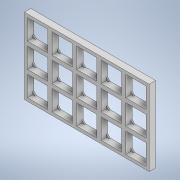
# Autodesk Inventor part: Cherry_Switch_Alignment_Jig
Saved by Autodesk Inventor 2022.2 (Build 262287000, 287)
## iProperties
Created: 2022-12-30
Part Number: Cherry_Switch_Alignment_Jig
Material: Generisch
Document SubType Name: Modeling
Designer: Frederik
Density: 1 g/cm^3
Appearance: Vorgabe
Author: Frederik
Autodesk Inventor part; units mm, degrees
ref_plane "YZ Plane" through (0, 0, 0) normal (1, 0, 0) x (0, 1, 0)
ref_plane "XZ Plane" through (0, 0, 0) normal (0, 1, 0) x (-1, 0, 0)
ref_plane "XY Plane" through (0, 0, 0) normal (0, 0, 1) x (1, 0, 0)
sketch "Skizze1" plane through (0, 0, 0) normal (0, 0, 1) x (1, 0, 0)
  line L0 (0, 0) -> (15.6, 0) construction
  line L1 (15.6, 0) -> (15.6, 15.6) construction
  line L2 (15.6, 15.6) -> (0, 15.6) construction
  line L3 (0, 15.6) -> (0, 0) construction
  line L4 (-0.09, 15.69) -> (15.69, 15.69)
  line L5 (15.69, 15.69) -> (15.69, -0.09)
  line L6 (15.69, -0.09) -> (-0.09, -0.09)
  line L7 (-0.09, -0.09) -> (-0.09, 15.69)
  line L8 (1.91, 15.69) -> (-0.09, 13.69)
  line L9 (13.69, 15.69) -> (15.69, 13.69)
  line L10 (15.69, 1.91) -> (13.69, -0.09)
  line L11 (1.91, -0.09) -> (-0.09, 1.91)
  line L12 (-0.09, -0.09) -> (15.69, 15.69) construction
  line L13 (15.69, -0.09) -> (-0.09, 15.69) construction
  line L14 (-1.725, 17.325) -> (17.325, 17.325)
  line L15 (17.325, 17.325) -> (17.325, -1.725)
  line L16 (17.325, -1.725) -> (-1.725, -1.725)
  line L17 (-1.725, -1.725) -> (-1.725, 17.325)
  point P0 (7.8, 7.8)
  point P1 (7.8, 7.8)
  dimension "d0" = 15.6
  dimension "d1" = 15.6
  dimension "d2" = 0.09
  dimension "d3" = 2
  dimension "d4" = 2
  dimension "d5" = 2
  dimension "d6" = 2
  dimension "d7" = 2
  dimension "d8" = 2
  dimension "d9" = 2
  dimension "d10" = 2
  dimension "d11" = 9.525
  constraints: 36 end point, 9 point on line, 6 parallel, 4 perpendicular, 2 midpoint, 1 horizontal, 6 other
  measures "d0" distance of L1.end L2.end
  measures "d1" distance of L0.end L1.end
  measures "d2" distance between parallel lines of L2 L4
  measures "d3" distance from line of L7 L8.start
  measures "d4" distance from line of L4 L8.end
  measures "d5" distance from line of L5 L9.start
  measures "d6" distance from line of L4 L9.end
  measures "d7" distance from line of L6 L10.start
  measures "d8" distance from line of L5 L10.end
  measures "d9" distance from line of L6 L11.end
  measures "d10" distance from line of L7 L11.start
  measures "d11" distance from line of L17 point (7.8, 7.8)
extrude "Extrusion1" add sketch "Skizze1" along normal blind 1 contours L4 L8 L7 | L4 L5 L9 | L11 L6 L7 | L5 L6 L10 | L14 L15 L16 L17
sketch "Skizze2" plane through (0, 0, 1) normal (0, 0, 1) x (1, 0, 0)
  line L0 (-1.725, -1.725) -> (17.325, -1.725) projected
  line L1 (17.325, -1.725) -> (17.325, 17.325) projected
  line L2 (17.325, 17.325) -> (-1.725, 17.325) projected
  line L3 (-1.725, 17.325) -> (-1.725, -1.725) projected
  line L4 (-0.09, 13.69) -> (1.91, 15.69) projected
  line L5 (1.91, 15.69) -> (13.69, 15.69) projected
  line L6 (13.69, 15.69) -> (15.69, 13.69) projected
  line L7 (15.69, 13.69) -> (15.69, 1.91) projected
  line L8 (15.69, 1.91) -> (13.69, -0.09) projected
  line L9 (13.69, -0.09) -> (1.91, -0.09) projected
  line L10 (1.91, -0.09) -> (-0.09, 1.91) projected
  line L11 (-0.09, 1.91) -> (-0.09, 13.69) projected
  line L12 (1.91, 15.69) -> (13.69, 15.69) projected
  line L13 (1.91, 15.69) -> (-0.09, 15.69)
  line L14 (-0.09, 15.69) -> (-0.09, 13.69)
  line L15 (-0.09, 1.91) -> (-0.09, 13.69) projected
  line L16 (-0.09, 1.91) -> (-0.09, -0.09)
  line L17 (-0.09, -0.09) -> (1.91, -0.09)
  line L18 (13.69, -0.09) -> (1.91, -0.09) projected
  line L19 (13.69, -0.09) -> (15.69, -0.09)
  line L20 (15.69, 1.91) -> (13.69, -0.09) projected
  line L21 (15.69, -0.09) -> (15.69, 1.91)
  line L22 (15.69, 13.69) -> (15.69, 1.91) projected
  line L23 (15.69, 13.69) -> (15.69, 15.69)
  line L24 (13.69, 15.69) -> (15.69, 13.69) projected
  line L25 (15.69, 15.69) -> (13.69, 15.69)
  point P0 (0, 0)
  constraints: 16 end point, 3 perpendicular, 3 point on line, 1 collinear, 1 vertical
extrude "Extrusion2" add sketch "Skizze2" along normal blind 4
pattern_linear "Rechteckige Anordnung1" count 5 spacing 19.05 along (1, 0, 0) count 3 spacing 19.05 along (0, -1, 0)
sketch "Skizze3" plane through (0, 0, 5) normal (0, 0, 1) x (1, 0, 0)
  line L0 (93.525, 17.325) -> (-1.725, 17.325) projected
  line L1 (-1.725, 17.325) -> (-1.725, -39.825) projected
  line L2 (-0.09, 15.69) -> (15.69, 15.69) projected
  line L3 (15.69, 15.69) -> (15.69, -0.09) projected
  line L4 (15.69, -0.09) -> (-0.09, -0.09) projected
  line L5 (-0.09, -0.09) -> (-0.09, 15.69) projected
  line L6 (-1.725, -39.825) -> (93.525, -39.825) projected
  line L7 (93.525, -39.825) -> (93.525, 17.325) projected
  line L8 (18.96, 15.69) -> (34.74, 15.69) projected
  line L9 (34.74, 15.69) -> (34.74, -0.09) projected
  line L10 (34.74, -0.09) -> (18.96, -0.09) projected
  line L11 (18.96, -0.09) -> (18.96, 15.69) projected
  line L12 (38.01, 15.69) -> (53.79, 15.69) projected
  line L13 (53.79, 15.69) -> (53.79, -0.09) projected
  line L14 (53.79, -0.09) -> (38.01, -0.09) projected
  line L15 (38.01, -0.09) -> (38.01, 15.69) projected
  line L16 (57.06, 15.69) -> (72.84, 15.69) projected
  line L17 (72.84, 15.69) -> (72.84, -0.09) projected
  line L18 (72.84, -0.09) -> (57.06, -0.09) projected
  line L19 (57.06, -0.09) -> (57.06, 15.69) projected
  line L20 (76.11, 15.69) -> (91.89, 15.69) projected
  line L21 (91.89, 15.69) -> (91.89, -0.09) projected
  line L22 (91.89, -0.09) -> (76.11, -0.09) projected
  line L23 (76.11, -0.09) -> (76.11, 15.69) projected
  line L24 (18.96, -3.36) -> (34.74, -3.36) projected
  line L25 (34.74, -3.36) -> (34.74, -19.14) projected
  line L26 (34.74, -19.14) -> (18.96, -19.14) projected
  line L27 (18.96, -19.14) -> (18.96, -3.36) projected
  line L28 (-0.09, -3.36) -> (15.69, -3.36) projected
  line L29 (15.69, -3.36) -> (15.69, -19.14) projected
  line L30 (15.69, -19.14) -> (-0.09, -19.14) projected
  line L31 (-0.09, -19.14) -> (-0.09, -3.36) projected
  line L32 (38.01, -3.36) -> (53.79, -3.36) projected
  line L33 (53.79, -3.36) -> (53.79, -19.14) projected
  line L34 (53.79, -19.14) -> (38.01, -19.14) projected
  line L35 (38.01, -19.14) -> (38.01, -3.36) projected
  line L36 (57.06, -3.36) -> (72.84, -3.36) projected
  line L37 (72.84, -3.36) -> (72.84, -19.14) projected
  line L38 (72.84, -19.14) -> (57.06, -19.14) projected
  line L39 (57.06, -19.14) -> (57.06, -3.36) projected
  line L40 (76.11, -3.36) -> (91.89, -3.36) projected
  line L41 (91.89, -3.36) -> (91.89, -19.14) projected
  line L42 (91.89, -19.14) -> (76.11, -19.14) projected
  line L43 (76.11, -19.14) -> (76.11, -3.36) projected
  line L44 (-0.09, -22.41) -> (15.69, -22.41) projected
  line L45 (15.69, -22.41) -> (15.69, -38.19) projected
  line L46 (15.69, -38.19) -> (-0.09, -38.19) projected
  line L47 (-0.09, -38.19) -> (-0.09, -22.41) projected
  line L48 (18.96, -22.41) -> (34.74, -22.41) projected
  line L49 (34.74, -22.41) -> (34.74, -38.19) projected
  line L50 (34.74, -38.19) -> (18.96, -38.19) projected
  line L51 (18.96, -38.19) -> (18.96, -22.41) projected
  line L52 (38.01, -22.41) -> (53.79, -22.41) projected
  line L53 (53.79, -22.41) -> (53.79, -38.19) projected
  line L54 (53.79, -38.19) -> (38.01, -38.19) projected
  line L55 (38.01, -38.19) -> (38.01, -22.41) projected
  line L56 (57.06, -22.41) -> (72.84, -22.41) projected
  line L57 (72.84, -22.41) -> (72.84, -38.19) projected
  line L58 (72.84, -38.19) -> (57.06, -38.19) projected
  line L59 (57.06, -38.19) -> (57.06, -22.41) projected
  line L60 (76.11, -22.41) -> (91.89, -22.41) projected
  line L61 (91.89, -22.41) -> (91.89, -38.19) projected
  line L62 (91.89, -38.19) -> (76.11, -38.19) projected
  line L63 (76.11, -38.19) -> (76.11, -22.41) projected
  line L64 (93.525, 17.325) -> (-1.725, 17.325) projected
  line L65 (-1.725, 17.325) -> (-1.725, -39.825) projected
  line L66 (-1.725, -39.825) -> (93.525, -39.825) projected
  line L67 (93.525, -39.825) -> (93.525, 17.325) projected
  line L68 (-0.09, 15.69) -> (15.69, 15.69) projected
  line L69 (15.69, 15.69) -> (15.69, -0.09) projected
  line L70 (15.69, -0.09) -> (-0.09, -0.09) projected
  line L71 (-0.09, -0.09) -> (-0.09, 15.69) projected
  line L72 (-2.49, 18.09) -> (94.29, 18.09)
  line L73 (94.29, 18.09) -> (94.29, -40.59)
  line L74 (94.29, -40.59) -> (-2.49, -40.59)
  line L75 (-2.49, -40.59) -> (-2.49, 18.09)
  dimension "d26" = 0.765
  constraints: 8 end point, 3 other
  measures "d26" distance between parallel lines of L0 L72
extrude "Extrusion3" add sketch "Skizze3" against normal up to surface (5 mm away) contours L72 L73 L74 L75
equation "\"d1\" = d0"
equation "\"d2\" = clearance"
equation "\"d3\" = dLength"
equation "\"d4\" = dLength"
equation "\"d5\" = dLength"
equation "\"d6\" = dLength"
equation "\"d7\" = dLength"
equation "\"d8\" = dLength"
equation "\"d9\" = dLength"
equation "\"d10\" = dLength"
equation "\"d26\" = border"
equation "\"clearance\" = 0.09"
equation "\"dLength\" = 2"
equation "\"border\" = 0.765"
